Autodesk Fusion 360 part; units mm, degrees
note: some values were not read from the file. Chosen so that the rebuilt part matches the saved one: which face or edge a step refers to. Set by a fixed rule: which sketch regions a step uses.
(part 2 of 2)
equation "d242 = drawer_width"
equation "d243 = drawer_height - thickness"
equation "d244 = thickness"
equation "d248 = ( drawer_height - drawer_backDovetailWidth ) / 2 - drawer_backPinWidth"
equation "d250 = thickness"
equation "d251 = 90 deg + dovetail_angle"
equation "d252 = d192"
equation "d253 = drawer_backDovetailWidth"
equation "d255 = drawer_backPinWidth"
equation "d256 = -thickness"
equation "d295 = drawer_width - thickness"
equation "d296 = depth - 2 * thickness"
equation "d297 = thickness"
equation "d322 = drawer_reveal"
equation "d335 = -thickness"
equation "d337 = -depth * 0.75"
equation "d340 = pull_width"
equation "d341 = pull_length + thickness"
equation "d342 = 90 deg - dovetail_angle"
equation "d343 = d342"
equation "d344 = thickness"
equation "d346 = pull_thickness"
equation "d348 = ( 1 / 32 ) * 1 in"
equation "d436 = drawer_reveal"
equation "d449 = -depth * 0.75"
equation "chamfer = ( 1 / 16 ) * 1 in"
equation "d457 = chamfer"
equation "d458 = chamfer"
equation "d459 = chamfer"
equation "d460 = chamfer"
equation "d461 = thickness"
equation "d462 = thickness * 0.8"
equation "d463 = wedge_thickness"
